Autodesk Fusion 360 part; units mm, degrees
(part 2 of 7)
  line L507 (63.4211, -56.2632) -> (63.3407, -56.2797)
  line L508 (63.3407, -56.2797) -> (63.3132, -56.4089)
  line L509 (63.3132, -56.4089) -> (63.2875, -56.5384)
  line L510 (63.2875, -56.5384) -> (63.2634, -56.6683)
  line L511 (63.2634, -56.6683) -> (63.3314, -56.7143)
  line L512 (63.3314, -56.7143) -> (63.3997, -56.7585)
  line L513 (63.3997, -56.7585) -> (63.4685, -56.801)
  line L514 (63.4685, -56.801) -> (63.5377, -56.8416)
  line L515 (63.5377, -56.8416) -> (63.6073, -56.8801)
  line L516 (63.6073, -56.8801) -> (63.6773, -56.9167)
  line L517 (63.6773, -56.9167) -> (63.7477, -56.951)
  line L518 (63.7477, -56.951) -> (63.8185, -56.9829)
  line L519 (63.8185, -56.9829) -> (63.8898, -57.0123)
  line L520 (63.8898, -57.0123) -> (63.9616, -57.0387)
  line L521 (63.9616, -57.0387) -> (64.0339, -57.0615)
  line L522 (64.0339, -57.0615) -> (64.107, -57.0789)
  line L523 (64.107, -57.0789) -> (64.5136, -57.1395)
  line L524 (64.5136, -57.1395) -> (64.4846, -57.3519)
  line L525 (64.4846, -57.3519) -> (64.461, -57.565)
  line L526 (64.461, -57.565) -> (64.4426, -57.7785)
  line L527 (64.4426, -57.7785) -> (64.4296, -57.9925)
  line L528 (64.4296, -57.9925) -> (64.019, -57.9726)
  line L529 (64.019, -57.9726) -> (63.9439, -57.9754)
  line L530 (63.9439, -57.9754) -> (63.8685, -57.9837)
  line L531 (63.8685, -57.9837) -> (63.793, -57.9956)
  line L532 (63.793, -57.9956) -> (63.7173, -58.0105)
  line L533 (63.7173, -58.0105) -> (63.6416, -58.028)
  line L534 (63.6416, -58.028) -> (63.5659, -58.0479)
  line L535 (63.5659, -58.0479) -> (63.4901, -58.0701)
  line L536 (63.4901, -58.0701) -> (63.4143, -58.0944)
  line L537 (63.4143, -58.0944) -> (63.3385, -58.1207)
  line L538 (63.3385, -58.1207) -> (63.2628, -58.1489)
  line L539 (63.2628, -58.1489) -> (63.1871, -58.1789)
  line L540 (63.1871, -58.1789) -> (63.1115, -58.2108)
  line L541 (63.1115, -58.2108) -> (63.1097, -58.3429)
  line L542 (63.1097, -58.3429) -> (63.1097, -58.4749)
  line L543 (63.1097, -58.4749) -> (63.1115, -58.607)
  line L544 (63.1115, -58.607) -> (63.1871, -58.6389)
  line L545 (63.1871, -58.6389) -> (63.2628, -58.6689)
  line L546 (63.2628, -58.6689) -> (63.3385, -58.6971)
  line L547 (63.3385, -58.6971) -> (63.4143, -58.7234)
  line L548 (63.4143, -58.7234) -> (63.4901, -58.7477)
  line L549 (63.4901, -58.7477) -> (63.5659, -58.7699)
  line L550 (63.5659, -58.7699) -> (63.6416, -58.7898)
  line L551 (63.6416, -58.7898) -> (63.7173, -58.8073)
  line L552 (63.7173, -58.8073) -> (63.793, -58.8222)
  line L553 (63.793, -58.8222) -> (63.8685, -58.8341)
  line L554 (63.8685, -58.8341) -> (63.9439, -58.8424)
  line L555 (63.9439, -58.8424) -> (64.019, -58.8452)
  line L556 (64.019, -58.8452) -> (64.4296, -58.8253)
  line L557 (64.4296, -58.8253) -> (64.4426, -59.0393)
  line L558 (64.4426, -59.0393) -> (64.461, -59.2528)
  line L559 (64.461, -59.2528) -> (64.4846, -59.4659)
  line L560 (64.4846, -59.4659) -> (64.5136, -59.6783)
  line L561 (64.5136, -59.6783) -> (64.107, -59.7389)
  line L562 (64.107, -59.7389) -> (64.0339, -59.7563)
  line L563 (64.0339, -59.7563) -> (63.9616, -59.7791)
  line L564 (63.9616, -59.7791) -> (63.8898, -59.8055)
  line L565 (63.8898, -59.8055) -> (63.8185, -59.8349)
  line L566 (63.8185, -59.8349) -> (63.7477, -59.8668)
  line L567 (63.7477, -59.8668) -> (63.6773, -59.9011)
  line L568 (63.6773, -59.9011) -> (63.6073, -59.9377)
  line L569 (63.6073, -59.9377) -> (63.5377, -59.9762)
  line L570 (63.5377, -59.9762) -> (63.4685, -60.0168)
  line L571 (63.4685, -60.0168) -> (63.3997, -60.0593)
  line L572 (63.3997, -60.0593) -> (63.3314, -60.1035)
  line L573 (63.3314, -60.1035) -> (63.2634, -60.1495)
  line L574 (63.2634, -60.1495) -> (63.2875, -60.2794)
  line L575 (63.2875, -60.2794) -> (63.3132, -60.4089)
  line L576 (63.3132, -60.4089) -> (63.3407, -60.5381)
  line L577 (63.3407, -60.5381) -> (63.4211, -60.5546)
  line L578 (63.4211, -60.5546) -> (63.5012, -60.5693)
  line L579 (63.5012, -60.5693) -> (63.581, -60.5822)
  line L580 (63.581, -60.5822) -> (63.6604, -60.5932)
  line L581 (63.6604, -60.5932) -> (63.7395, -60.6022)
  line L582 (63.7395, -60.6022) -> (63.8181, -60.6092)
  line L583 (63.8181, -60.6092) -> (63.8963, -60.614)
  line L584 (63.8963, -60.614) -> (63.974, -60.6164)
  line L585 (63.974, -60.6164) -> (64.0511, -60.6162)
  line L586 (64.0511, -60.6162) -> (64.1275, -60.6131)
  line L587 (64.1275, -60.6131) -> (64.203, -60.6065)
  line L588 (64.203, -60.6065) -> (64.2773, -60.5947)
  line L589 (64.2773, -60.5947) -> (64.6761, -60.4951)
  line L590 (64.6761, -60.4951) -> (64.7306, -60.7024)
  line L591 (64.7306, -60.7024) -> (64.7903, -60.9083)
  line L592 (64.7903, -60.9083) -> (64.855, -61.1126)
  line L593 (64.855, -61.1126) -> (64.9249, -61.3152)
  line L594 (64.9249, -61.3152) -> (64.538, -61.454)
  line L595 (64.538, -61.454) -> (64.4696, -61.4854)
  line L596 (64.4696, -61.4854) -> (64.4031, -61.5218)
  line L597 (64.4031, -61.5218) -> (64.3379, -61.5617)
  line L598 (64.3379, -61.5617) -> (64.2737, -61.6044)
  line L599 (64.2737, -61.6044) -> (64.2105, -61.6496)
  line L600 (64.2105, -61.6496) -> (64.1481, -61.697)
  line L601 (64.1481, -61.697) -> (64.0866, -61.7465)
  line L602 (64.0866, -61.7465) -> (64.0259, -61.7979)
  line L603 (64.0259, -61.7979) -> (63.9659, -61.8512)
  line L604 (63.9659, -61.8512) -> (63.9067, -61.9062)
  line L605 (63.9067, -61.9062) -> (63.8483, -61.963)
  line L606 (63.8483, -61.963) -> (63.7907, -62.0214)
  line L607 (63.7907, -62.0214) -> (63.8396, -62.144)
  line L608 (63.8396, -62.144) -> (63.8901, -62.266)
  line L609 (63.8901, -62.266) -> (63.9423, -62.3874)
  line L610 (63.9423, -62.3874) -> (64.0243, -62.3879)
  line L611 (64.0243, -62.3879) -> (64.1058, -62.3867)
  line L612 (64.1058, -62.3867) -> (64.1865, -62.3838)
  line L613 (64.1865, -62.3838) -> (64.2666, -62.3791)
  line L614 (64.2666, -62.3791) -> (64.3459, -62.3725)
  line L615 (64.3459, -62.3725) -> (64.4244, -62.364)
  line L616 (64.4244, -62.364) -> (64.502, -62.3534)
  line L617 (64.502, -62.3534) -> (64.5787, -62.3406)
  line L618 (64.5787, -62.3406) -> (64.6542, -62.3254)
  line L619 (64.6542, -62.3254) -> (64.7286, -62.3075)
  line L620 (64.7286, -62.3075) -> (64.8014, -62.2863)
  line L621 (64.8014, -62.2863) -> (64.8719, -62.2601)
  line L622 (64.8719, -62.2601) -> (65.2436, -62.0847)
  line L623 (65.2436, -62.0847) -> (65.3375, -62.2773)
  line L624 (65.3375, -62.2773) -> (65.4362, -62.4676)
  line L625 (65.4362, -62.4676) -> (65.5396, -62.6554)
  line L626 (65.5396, -62.6554) -> (65.6476, -62.8405)
  line L627 (65.6476, -62.8405) -> (65.2952, -63.0521)
  line L628 (65.2952, -63.0521) -> (65.2343, -63.0962)
  line L629 (65.2343, -63.0962) -> (65.1762, -63.145)
  line L630 (65.1762, -63.145) -> (65.12, -63.1968)
  line L631 (65.12, -63.1968) -> (65.0654, -63.2512)
  line L632 (65.0654, -63.2512) -> (65.0122, -63.3078)
  line L633 (65.0122, -63.3078) -> (64.9602, -63.3665)
  line L634 (64.9602, -63.3665) -> (64.9096, -63.427)
  line L635 (64.9096, -63.427) -> (64.86, -63.4893)
  line L636 (64.86, -63.4893) -> (64.8116, -63.5532)
  line L637 (64.8116, -63.5532) -> (64.7643, -63.6188)
  line L638 (64.7643, -63.6188) -> (64.7181, -63.6858)
  line L639 (64.7181, -63.6858) -> (64.6729, -63.7544)
  line L640 (64.6729, -63.7544) -> (64.7448, -63.8651)
  line L641 (64.7448, -63.8651) -> (64.8182, -63.9749)
  line L642 (64.8182, -63.9749) -> (64.893, -64.0838)
  line L643 (64.893, -64.0838) -> (64.9736, -64.0683)
  line L644 (64.9736, -64.0683) -> (65.0533, -64.0512)
  line L645 (65.0533, -64.0512) -> (65.1319, -64.0326)
  line L646 (65.1319, -64.0326) -> (65.2095, -64.0123)
  line L647 (65.2095, -64.0123) -> (65.286, -63.9904)
  line L648 (65.286, -63.9904) -> (65.3613, -63.9667)
  line L649 (65.3613, -63.9667) -> (65.4354, -63.9412)
  line L650 (65.4354, -63.9412) -> (65.5081, -63.9137)
  line L651 (65.5081, -63.9137) -> (65.5792, -63.8841)
  line L652 (65.5792, -63.8841) -> (65.6486, -63.852)
  line L653 (65.6486, -63.852) -> (65.7159, -63.817)
  line L654 (65.7159, -63.817) -> (65.78, -63.7776)
  line L655 (65.78, -63.7776) -> (66.1103, -63.533)
  line L656 (66.1103, -63.533) -> (66.24, -63.7036)
  line L657 (66.24, -63.7036) -> (66.3739, -63.871)
  line L658 (66.3739, -63.871) -> (66.5119, -64.035)
  line L659 (66.5119, -64.035) -> (66.654, -64.1955)
  line L660 (66.654, -64.1955) -> (66.3496, -64.4718)
  line L661 (66.3496, -64.4718) -> (66.2985, -64.5269)
  line L662 (66.2985, -64.5269) -> (66.2511, -64.5861)
  line L663 (66.2511, -64.5861) -> (66.2061, -64.6479)
  line L664 (66.2061, -64.6479) -> (66.1631, -64.7119)
  line L665 (66.1631, -64.7119) -> (66.122, -64.7778)
  line L666 (66.122, -64.7778) -> (66.0825, -64.8455)
  line L667 (66.0825, -64.8455) -> (66.0446, -64.9147)
  line L668 (66.0446, -64.9147) -> (66.0081, -64.9855)
  line L669 (66.0081, -64.9855) -> (65.9731, -65.0576)
  line L670 (65.9731, -65.0576) -> (65.9395, -65.1311)
  line L671 (65.9395, -65.1311) -> (65.9073, -65.2059)
  line L672 (65.9073, -65.2059) -> (65.8764, -65.2819)
  line L673 (65.8764, -65.2819) -> (65.9685, -65.3766)
  line L674 (65.9685, -65.3766) -> (66.0619, -65.4699)
  line L675 (66.0619, -65.4699) -> (66.1565, -65.5621)
  line L676 (66.1565, -65.5621) -> (66.2325, -65.5311)
  line L677 (66.2325, -65.5311) -> (66.3073, -65.4989)
  line L678 (66.3073, -65.4989) -> (66.3808, -65.4653)
  line L679 (66.3808, -65.4653) -> (66.4529, -65.4303)
  line L680 (66.4529, -65.4303) -> (66.5237, -65.3939)
  line L681 (66.5237, -65.3939) -> (66.593, -65.3559)
  line L682 (66.593, -65.3559) -> (66.6606, -65.3165)
  line L683 (66.6606, -65.3165) -> (66.7265, -65.2753)
  line L684 (66.7265, -65.2753) -> (66.7905, -65.2324)
  line L685 (66.7905, -65.2324) -> (66.8524, -65.1874)
  line L686 (66.8524, -65.1874) -> (66.9115, -65.1399)
  line L687 (66.9115, -65.1399) -> (66.9666, -65.0888)
  line L688 (66.9666, -65.0888) -> (67.2429, -64.7844)
  line L689 (67.2429, -64.7844) -> (67.4034, -64.9265)
  line L690 (67.4034, -64.9265) -> (67.5674, -65.0645)
  line L691 (67.5674, -65.0645) -> (67.7348, -65.1984)
  line L692 (67.7348, -65.1984) -> (67.9054, -65.3281)
  line L693 (67.9054, -65.3281) -> (67.6608, -65.6585)
  line L694 (67.6608, -65.6585) -> (67.6214, -65.7225)
  line L695 (67.6214, -65.7225) -> (67.5864, -65.7898)
  line L696 (67.5864, -65.7898) -> (67.5543, -65.8592)
  line L697 (67.5543, -65.8592) -> (67.5247, -65.9303)
  line L698 (67.5247, -65.9303) -> (67.4972, -66.003)
  line L699 (67.4972, -66.003) -> (67.4717, -66.0771)
  line L700 (67.4717, -66.0771) -> (67.448, -66.1524)
  line L701 (67.448, -66.1524) -> (67.4261, -66.2289)
  line L702 (67.4261, -66.2289) -> (67.4058, -66.3065)
  line L703 (67.4058, -66.3065) -> (67.3872, -66.3852)
  line L704 (67.3872, -66.3852) -> (67.3702, -66.4648)
  line L705 (67.3702, -66.4648) -> (67.3547, -66.5454)
  line L706 (67.3547, -66.5454) -> (67.4635, -66.6202)
  line L707 (67.4635, -66.6202) -> (67.5733, -66.6936)
  line L708 (67.5733, -66.6936) -> (67.6841, -66.7655)
  line L709 (67.6841, -66.7655) -> (67.7526, -66.7203)
  line L710 (67.7526, -66.7203) -> (67.8196, -66.6741)
  line L711 (67.8196, -66.6741) -> (67.8852, -66.6268)
  line L712 (67.8852, -66.6268) -> (67.9491, -66.5784)
  line L713 (67.9491, -66.5784) -> (68.0114, -66.5289)
  line L714 (68.0114, -66.5289) -> (68.0719, -66.4782)
  line L715 (68.0719, -66.4782) -> (68.1306, -66.4263)
  line L716 (68.1306, -66.4263) -> (68.1872, -66.373)
  line L717 (68.1872, -66.373) -> (68.2416, -66.3184)
  line L718 (68.2416, -66.3184) -> (68.2935, -66.2622)
  line L719 (68.2935, -66.2622) -> (68.3422, -66.2041)
  line L720 (68.3422, -66.2041) -> (68.3863, -66.1432)
  line L721 (68.3863, -66.1432) -> (68.5979, -65.7908)
  line L722 (68.5979, -65.7908) -> (68.783, -65.8989)
  line L723 (68.783, -65.8989) -> (68.9708, -66.0022)
  line L724 (68.9708, -66.0022) -> (69.1611, -66.1009)
  line L725 (69.1611, -66.1009) -> (69.3538, -66.1948)
  line L726 (69.3538, -66.1948) -> (69.1783, -66.5665)
  line L727 (69.1783, -66.5665) -> (69.1521, -66.6371)
  line L728 (69.1521, -66.6371) -> (69.1309, -66.7099)
  line L729 (69.1309, -66.7099) -> (69.113, -66.7842)
  line L730 (69.113, -66.7842) -> (69.0978, -66.8598)
  line L731 (69.0978, -66.8598) -> (69.085, -66.9364)
  line L732 (69.085, -66.9364) -> (69.0745, -67.014)
  line L733 (69.0745, -67.014) -> (69.0659, -67.0925)
  line L734 (69.0659, -67.0925) -> (69.0594, -67.1718)
  line L735 (69.0594, -67.1718) -> (69.0546, -67.2519)
  line L736 (69.0546, -67.2519) -> (69.0517, -67.3327)
  line L737 (69.0517, -67.3327) -> (69.0505, -67.4141)
  line L738 (69.0505, -67.4141) -> (69.0511, -67.4962)
  line L739 (69.0511, -67.4962) -> (69.1724, -67.5483)
  line L740 (69.1724, -67.5483) -> (69.2944, -67.5989)
  line L741 (69.2944, -67.5989) -> (69.4171, -67.6478)
  line L742 (69.4171, -67.6478) -> (69.4755, -67.5901)
  line L743 (69.4755, -67.5901) -> (69.5322, -67.5317)
  line L744 (69.5322, -67.5317) -> (69.5873, -67.4725)
  line L745 (69.5873, -67.4725) -> (69.6405, -67.4126)
  line L746 (69.6405, -67.4126) -> (69.692, -67.3518)
  line L747 (69.692, -67.3518) -> (69.7414, -67.2903)
  line L748 (69.7414, -67.2903) -> (69.7888, -67.2279)
  line L749 (69.7888, -67.2279) -> (69.834, -67.1647)
  line L750 (69.834, -67.1647) -> (69.8767, -67.1005)
  line L751 (69.8767, -67.1005) -> (69.9166, -67.0353)
  line L752 (69.9166, -67.0353) -> (69.9531, -66.9688)
  line L753 (69.9531, -66.9688) -> (69.9844, -66.9005)
  line L754 (69.9844, -66.9005) -> (70.1232, -66.5135)
  line L755 (70.1232, -66.5135) -> (70.3258, -66.5834)
  line L756 (70.3258, -66.5834) -> (70.5302, -66.6482)
  line L757 (70.5302, -66.6482) -> (70.7361, -66.7078)
  line L758 (70.7361, -66.7078) -> (70.9434, -66.7623)
  line L759 (70.9434, -66.7623) -> (70.8438, -67.1611)
  line L760 (70.8438, -67.1611) -> (70.8319, -67.2354)
  line L761 (70.8319, -67.2354) -> (70.8253, -67.3109)
  line L762 (70.8253, -67.3109) -> (70.8222, -67.3873)
  line L763 (70.8222, -67.3873) -> (70.822, -67.4644)
  line L764 (70.822, -67.4644) -> (70.8245, -67.5421)
  line L765 (70.8245, -67.5421) -> (70.8292, -67.6203)
  line L766 (70.8292, -67.6203) -> (70.8362, -67.6989)
  line L767 (70.8362, -67.6989) -> (70.8452, -67.778)
  line L768 (70.8452, -67.778) -> (70.8562, -67.8574)
  line L769 (70.8562, -67.8574) -> (70.8691, -67.9372)
  line L770 (70.8691, -67.9372) -> (70.8838, -68.0173)
  line L771 (70.8838, -68.0173) -> (70.9003, -68.0977)
  line L772 (70.9003, -68.0977) -> (71.0295, -68.1252)
  line L773 (71.0295, -68.1252) -> (71.159, -68.151)
  line L774 (71.159, -68.151) -> (71.2889, -68.175)
  line L775 (71.2889, -68.175) -> (71.3349, -68.107)
  line L776 (71.3349, -68.107) -> (71.3792, -68.0387)
  line L777 (71.3792, -68.0387) -> (71.4216, -67.9699)
  line L778 (71.4216, -67.9699) -> (71.4622, -67.9007)
  line L779 (71.4622, -67.9007) -> (71.5008, -67.8311)
  line L780 (71.5008, -67.8311) -> (71.5373, -67.7611)
  line L781 (71.5373, -67.7611) -> (71.5716, -67.6907)
  line L782 (71.5716, -67.6907) -> (71.6036, -67.6199)
  line L783 (71.6036, -67.6199) -> (71.6329, -67.5486)
  line L784 (71.6329, -67.5486) -> (71.6593, -67.4768)
  line L785 (71.6593, -67.4768) -> (71.6821, -67.4045)
  line L786 (71.6821, -67.4045) -> (71.6996, -67.3314)
  line L787 (71.6996, -67.3314) -> (71.7602, -66.9248)
  line L788 (71.7602, -66.9248) -> (71.9726, -66.9538)
  line L789 (71.9726, -66.9538) -> (72.1856, -66.9774)
  line L790 (72.1856, -66.9774) -> (72.3992, -66.9958)
  line L791 (72.3992, -66.9958) -> (72.6131, -67.0088)
  line L792 (72.6131, -67.0088) -> (72.5932, -67.4194)
  line L793 (72.5932, -67.4194) -> (72.5961, -67.4945)
  line L794 (72.5961, -67.4945) -> (72.6043, -67.5699)
  line L795 (72.6043, -67.5699) -> (72.6162, -67.6454)
  line L796 (72.6162, -67.6454) -> (72.6311, -67.7211)
  line L797 (72.6311, -67.7211) -> (72.6486, -67.7968)
  line L798 (72.6486, -67.7968) -> (72.6686, -67.8725)
  line L799 (72.6686, -67.8725) -> (72.6907, -67.9483)
  line L800 (72.6907, -67.9483) -> (72.715, -68.0241)
  line L801 (72.715, -68.0241) -> (72.7413, -68.0999)
  line L802 (72.7413, -68.0999) -> (72.7695, -68.1756)
  line L803 (72.7695, -68.1756) -> (72.7996, -68.2513)
  line L804 (72.7996, -68.2513) -> (72.8314, -68.3269)
  line L805 (72.8314, -68.3269) -> (72.9635, -68.3287)
  line L806 (72.9635, -68.3287) -> (73.0956, -68.3287)
  line L807 (73.0956, -68.3287) -> (73.2276, -68.3269)
  line L808 (73.2276, -68.3269) -> (73.2595, -68.2513)
  line L809 (73.2595, -68.2513) -> (73.2896, -68.1756)
  line L810 (73.2896, -68.1756) -> (73.3178, -68.0999)
  line L811 (73.3178, -68.0999) -> (73.3441, -68.0241)
  line L812 (73.3441, -68.0241) -> (73.3683, -67.9483)
  line L813 (73.3683, -67.9483) -> (73.3905, -67.8725)
  line L814 (73.3905, -67.8725) -> (73.4104, -67.7968)
  line L815 (73.4104, -67.7968) -> (73.4279, -67.7211)
  line L816 (73.4279, -67.7211) -> (73.4428, -67.6454)
  line L817 (73.4428, -67.6454) -> (73.4547, -67.5699)
  line L818 (73.4547, -67.5699) -> (73.463, -67.4945)
  line L819 (73.463, -67.4945) -> (73.4658, -67.4194)
  line L820 (73.4658, -67.4194) -> (73.4459, -67.0088)
  line L821 (73.4459, -67.0088) -> (73.6599, -66.9958)
  line L822 (73.6599, -66.9958) -> (73.8734, -66.9774)
  line L823 (73.8734, -66.9774) -> (74.0865, -66.9538)
  line L824 (74.0865, -66.9538) -> (74.2989, -66.9248)
  line L825 (74.2989, -66.9248) -> (74.3595, -67.3314)
  line L826 (74.3595, -67.3314) -> (74.3769, -67.4045)
  line L827 (74.3769, -67.4045) -> (74.3997, -67.4768)
  line L828 (74.3997, -67.4768) -> (74.4261, -67.5486)
  line L829 (74.4261, -67.5486) -> (74.4555, -67.6199)
  line L830 (74.4555, -67.6199) -> (74.4874, -67.6907)
  line L831 (74.4874, -67.6907) -> (74.5218, -67.7611)
  line L832 (74.5218, -67.7611) -> (74.5583, -67.8311)
  line L833 (74.5583, -67.8311) -> (74.5969, -67.9007)
  line L834 (74.5969, -67.9007) -> (74.6374, -67.9699)
  line L835 (74.6374, -67.9699) -> (74.6799, -68.0387)
  line L836 (74.6799, -68.0387) -> (74.7241, -68.107)
  line L837 (74.7241, -68.107) -> (74.7702, -68.175)
  line L838 (74.7702, -68.175) -> (74.9, -68.151)
  line L839 (74.9, -68.151) -> (75.0295, -68.1252)
  line L840 (75.0295, -68.1252) -> (75.1587, -68.0977)
  line L841 (75.1587, -68.0977) -> (75.1752, -68.0173)
  line L842 (75.1752, -68.0173) -> (75.19, -67.9372)
  line L843 (75.19, -67.9372) -> (75.2028, -67.8574)
  line L844 (75.2028, -67.8574) -> (75.2138, -67.778)
  line L845 (75.2138, -67.778) -> (75.2229, -67.6989)
  line L846 (75.2229, -67.6989) -> (75.2298, -67.6203)
  line L847 (75.2298, -67.6203) -> (75.2346, -67.5421)
  line L848 (75.2346, -67.5421) -> (75.237, -67.4644)
  line L849 (75.237, -67.4644) -> (75.2368, -67.3873)
  line L850 (75.2368, -67.3873) -> (75.2338, -67.3109)
  line L851 (75.2338, -67.3109) -> (75.2272, -67.2354)
  line L852 (75.2272, -67.2354) -> (75.2153, -67.1611)
  line L853 (75.2153, -67.1611) -> (75.1157, -66.7623)
  line L854 (75.1157, -66.7623) -> (75.323, -66.7078)
  line L855 (75.323, -66.7078) -> (75.5289, -66.6482)
  line L856 (75.5289, -66.6482) -> (75.7332, -66.5834)
  line L857 (75.7332, -66.5834) -> (75.9359, -66.5135)
  line L858 (75.9359, -66.5135) -> (76.0746, -66.9005)
  line L859 (76.0746, -66.9005) -> (76.106, -66.9688)
  line L860 (76.106, -66.9688) -> (76.1425, -67.0353)
  line L861 (76.1425, -67.0353) -> (76.1824, -67.1005)
  line L862 (76.1824, -67.1005) -> (76.2251, -67.1647)
  line L863 (76.2251, -67.1647) -> (76.2702, -67.2279)
  line L864 (76.2702, -67.2279) -> (76.3176, -67.2903)
  line L865 (76.3176, -67.2903) -> (76.3671, -67.3518)
  line L866 (76.3671, -67.3518) -> (76.4185, -67.4126)
  line L867 (76.4185, -67.4126) -> (76.4718, -67.4725)
  line L868 (76.4718, -67.4725) -> (76.5268, -67.5317)
  line L869 (76.5268, -67.5317) -> (76.5836, -67.5901)
  line L870 (76.5836, -67.5901) -> (76.642, -67.6478)
  line L871 (76.642, -67.6478) -> (76.7647, -67.5989)
  line L872 (76.7647, -67.5989) -> (76.8867, -67.5483)
  line L873 (76.8867, -67.5483) -> (77.008, -67.4962)
  line L874 (77.008, -67.4962) -> (77.0085, -67.4141)
  line L875 (77.0085, -67.4141) -> (77.0073, -67.3327)
  line L876 (77.0073, -67.3327) -> (77.0044, -67.2519)
  line L877 (77.0044, -67.2519) -> (76.9997, -67.1718)
  line L878 (76.9997, -67.1718) -> (76.9931, -67.0925)
  line L879 (76.9931, -67.0925) -> (76.9846, -67.014)
  line L880 (76.9846, -67.014) -> (76.974, -66.9364)
  line L881 (76.974, -66.9364) -> (76.9612, -66.8598)
  line L882 (76.9612, -66.8598) -> (76.946, -66.7842)
  line L883 (76.946, -66.7842) -> (76.9281, -66.7099)
  line L884 (76.9281, -66.7099) -> (76.9069, -66.6371)
  line L885 (76.9069, -66.6371) -> (76.8808, -66.5665)
  line L886 (76.8808, -66.5665) -> (76.7053, -66.1948)
  line L887 (76.7053, -66.1948) -> (76.898, -66.1009)
  line L888 (76.898, -66.1009) -> (77.0882, -66.0022)
  line L889 (77.0882, -66.0022) -> (77.276, -65.8989)
  line L890 (77.276, -65.8989) -> (77.4612, -65.7908)
  line L891 (77.4612, -65.7908) -> (77.6727, -66.1432)
  line L892 (77.6727, -66.1432) -> (77.7168, -66.2041)
  line L893 (77.7168, -66.2041) -> (77.7656, -66.2622)
  line L894 (77.7656, -66.2622) -> (77.8174, -66.3184)
  line L895 (77.8174, -66.3184) -> (77.8718, -66.373)
  line L896 (77.8718, -66.373) -> (77.9285, -66.4263)
  line L897 (77.9285, -66.4263) -> (77.9871, -66.4782)
  line L898 (77.9871, -66.4782) -> (78.0476, -66.5289)
  line L899 (78.0476, -66.5289) -> (78.1099, -66.5784)
  line L900 (78.1099, -66.5784) -> (78.1739, -66.6268)
  line L901 (78.1739, -66.6268) -> (78.2394, -66.6741)
  line L902 (78.2394, -66.6741) -> (78.3065, -66.7203)
  line L903 (78.3065, -66.7203) -> (78.375, -66.7655)
  line L904 (78.375, -66.7655) -> (78.4858, -66.6936)
  line L905 (78.4858, -66.6936) -> (78.5956, -66.6202)
  line L906 (78.5956, -66.6202) -> (78.7044, -66.5454)
  line L907 (78.7044, -66.5454) -> (78.6889, -66.4648)
  line L908 (78.6889, -66.4648) -> (78.6718, -66.3852)
  line L909 (78.6718, -66.3852) -> (78.6532, -66.3065)
  line L910 (78.6532, -66.3065) -> (78.633, -66.2289)
  line L911 (78.633, -66.2289) -> (78.611, -66.1524)
  line L912 (78.611, -66.1524) -> (78.5874, -66.0771)
  line L913 (78.5874, -66.0771) -> (78.5619, -66.003)
  line L914 (78.5619, -66.003) -> (78.5344, -65.9303)
  line L915 (78.5344, -65.9303) -> (78.5047, -65.8592)
  line L916 (78.5047, -65.8592) -> (78.4726, -65.7898)
  line L917 (78.4726, -65.7898) -> (78.4376, -65.7225)
  line L918 (78.4376, -65.7225) -> (78.3982, -65.6585)
  line L919 (78.3982, -65.6585) -> (78.1536, -65.3281)
  line L920 (78.1536, -65.3281) -> (78.3243, -65.1984)
  line L921 (78.3243, -65.1984) -> (78.4916, -65.0645)
  line L922 (78.4916, -65.0645) -> (78.6556, -64.9265)
  line L923 (78.6556, -64.9265) -> (78.8161, -64.7844)
  line L924 (78.8161, -64.7844) -> (79.0924, -65.0888)
  line L925 (79.0924, -65.0888) -> (79.1475, -65.1399)
  line L926 (79.1475, -65.1399) -> (79.2067, -65.1874)
  line L927 (79.2067, -65.1874) -> (79.2685, -65.2324)
  line L928 (79.2685, -65.2324) -> (79.3325, -65.2753)
  line L929 (79.3325, -65.2753) -> (79.3984, -65.3165)
  line L930 (79.3984, -65.3165) -> (79.4661, -65.3559)
  line L931 (79.4661, -65.3559) -> (79.5353, -65.3939)
  line L932 (79.5353, -65.3939) -> (79.6061, -65.4303)
  line L933 (79.6061, -65.4303) -> (79.6783, -65.4653)
  line L934 (79.6783, -65.4653) -> (79.7518, -65.4989)
  line L935 (79.7518, -65.4989) -> (79.8265, -65.5311)
  line L936 (79.8265, -65.5311) -> (79.9026, -65.5621)
  line L937 (79.9026, -65.5621) -> (79.9972, -65.4699)
  line L938 (79.9972, -65.4699) -> (80.0906, -65.3766)
  line L939 (80.0906, -65.3766) -> (80.1827, -65.2819)
  line L940 (80.1827, -65.2819) -> (80.1518, -65.2059)
  line L941 (80.1518, -65.2059) -> (80.1195, -65.1311)
  line L942 (80.1195, -65.1311) -> (80.0859, -65.0576)
  line L943 (80.0859, -65.0576) -> (80.0509, -64.9855)
  line L944 (80.0509, -64.9855) -> (80.0145, -64.9147)
  line L945 (80.0145, -64.9147) -> (79.9766, -64.8455)
  line L946 (79.9766, -64.8455) -> (79.9371, -64.7778)
  line L947 (79.9371, -64.7778) -> (79.8959, -64.7119)
  line L948 (79.8959, -64.7119) -> (79.853, -64.6479)
  line L949 (79.853, -64.6479) -> (79.808, -64.5861)
  line L950 (79.808, -64.5861) -> (79.7605, -64.5269)
  line L951 (79.7605, -64.5269) -> (79.7094, -64.4718)
  line L952 (79.7094, -64.4718) -> (79.405, -64.1955)
  line L953 (79.405, -64.1955) -> (79.5471, -64.035)
  line L954 (79.5471, -64.035) -> (79.6851, -63.871)
  line L955 (79.6851, -63.871) -> (79.8191, -63.7036)
  line L956 (79.8191, -63.7036) -> (79.9488, -63.533)
  line L957 (79.9488, -63.533) -> (80.2791, -63.7776)
  line L958 (80.2791, -63.7776) -> (80.3431, -63.817)
  line L959 (80.3431, -63.817) -> (80.4104, -63.852)
  line L960 (80.4104, -63.852) -> (80.4798, -63.8841)
  line L961 (80.4798, -63.8841) -> (80.551, -63.9137)
  line L962 (80.551, -63.9137) -> (80.6237, -63.9412)
  line L963 (80.6237, -63.9412) -> (80.6977, -63.9667)
  line L964 (80.6977, -63.9667) -> (80.773, -63.9904)
  line L965 (80.773, -63.9904) -> (80.8495, -64.0123)
  line L966 (80.8495, -64.0123) -> (80.9271, -64.0326)
  line L967 (80.9271, -64.0326) -> (81.0058, -64.0512)
  line L968 (81.0058, -64.0512) -> (81.0854, -64.0683)
  line L969 (81.0854, -64.0683) -> (81.166, -64.0838)
  line L970 (81.166, -64.0838) -> (81.2408, -63.9749)
  line L971 (81.2408, -63.9749) -> (81.3142, -63.8651)
  line L972 (81.3142, -63.8651) -> (81.3861, -63.7544)
  line L973 (81.3861, -63.7544) -> (81.3409, -63.6858)
  line L974 (81.3409, -63.6858) -> (81.2947, -63.6188)
  line L975 (81.2947, -63.6188) -> (81.2474, -63.5532)
  line L976 (81.2474, -63.5532) -> (81.199, -63.4893)
  line L977 (81.199, -63.4893) -> (81.1495, -63.427)
  line L978 (81.1495, -63.427) -> (81.0988, -63.3665)
  line L979 (81.0988, -63.3665) -> (81.0469, -63.3078)
  line L980 (81.0469, -63.3078) -> (80.9937, -63.2512)
  line L981 (80.9937, -63.2512) -> (80.939, -63.1968)
  line L982 (80.939, -63.1968) -> (80.8828, -63.145)
  line L983 (80.8828, -63.145) -> (80.8248, -63.0962)
  line L984 (80.8248, -63.0962) -> (80.7639, -63.0521)
  line L985 (80.7639, -63.0521) -> (80.4114, -62.8405)
  line L986 (80.4114, -62.8405) -> (80.5195, -62.6554)
  line L987 (80.5195, -62.6554) -> (80.6229, -62.4676)
  line L988 (80.6229, -62.4676) -> (80.7215, -62.2773)
  line L989 (80.7215, -62.2773) -> (80.8155, -62.0847)
  line L990 (80.8155, -62.0847) -> (81.1872, -62.2601)
  line L991 (81.1872, -62.2601) -> (81.2577, -62.2863)
  line L992 (81.2577, -62.2863) -> (81.3305, -62.3075)
  line L993 (81.3305, -62.3075) -> (81.4048, -62.3254)
  line L994 (81.4048, -62.3254) -> (81.4804, -62.3406)
  line L995 (81.4804, -62.3406) -> (81.557, -62.3534)
  line L996 (81.557, -62.3534) -> (81.6347, -62.364)
  line L997 (81.6347, -62.364) -> (81.7131, -62.3725)
  line L998 (81.7131, -62.3725) -> (81.7924, -62.3791)
  line L999 (81.7924, -62.3791) -> (81.8725, -62.3838)
  line L1000 (81.8725, -62.3838) -> (81.9533, -62.3867)
  line L1001 (81.9533, -62.3867) -> (82.0347, -62.3879)
  line L1002 (82.0347, -62.3879) -> (82.1168, -62.3874)
  line L1003 (82.1168, -62.3874) -> (82.1689, -62.266)
  line L1004 (82.1689, -62.266) -> (82.2195, -62.144)
  line L1005 (82.2195, -62.144) -> (82.2684, -62.0214)
  line L1006 (82.2684, -62.0214) -> (82.2107, -61.963)
  line L1007 (82.2107, -61.963) -> (82.1523, -61.9062)
  line L1008 (82.1523, -61.9062) -> (82.0931, -61.8512)
  line L1009 (82.0931, -61.8512) -> (82.0332, -61.7979)
  line L1010 (82.0332, -61.7979) -> (81.9725, -61.7465)
  line L1011 (81.9725, -61.7465) -> (81.9109, -61.697)
  line L1012 (81.9109, -61.697) -> (81.8486, -61.6496)
  line L1013 (81.8486, -61.6496) -> (81.7853, -61.6044)
  line L1014 (81.7853, -61.6044) -> (81.7211, -61.5617)
  line L1015 (81.7211, -61.5617) -> (81.6559, -61.5218)
  line L1016 (81.6559, -61.5218) -> (81.5894, -61.4854)
  line L1017 (81.5894, -61.4854) -> (81.5211, -61.454)
  line L1018 (81.5211, -61.454) -> (81.1342, -61.3152)
  line L1019 (81.1342, -61.3152) -> (81.204, -61.1126)
  line L1020 (81.204, -61.1126) -> (81.2688, -60.9083)
  line L1021 (81.2688, -60.9083) -> (81.3284, -60.7024)
  line L1022 (81.3284, -60.7024) -> (81.383, -60.4951)
  line L1023 (81.383, -60.4951) -> (81.7818, -60.5947)
  line L1024 (81.7818, -60.5947) -> (81.856, -60.6065)
  line L1025 (81.856, -60.6065) -> (81.9316, -60.6131)
  line L1026 (81.9316, -60.6131) -> (82.008, -60.6162)
  line L1027 (82.008, -60.6162) -> (82.085, -60.6164)
  line L1028 (82.085, -60.6164) -> (82.1627, -60.614)
  line L1029 (82.1627, -60.614) -> (82.2409, -60.6092)
  line L1030 (82.2409, -60.6092) -> (82.3195, -60.6022)
  line L1031 (82.3195, -60.6022) -> (82.3986, -60.5932)
  line L1032 (82.3986, -60.5932) -> (82.4781, -60.5822)
  line L1033 (82.4781, -60.5822) -> (82.5578, -60.5693)
  line L1034 (82.5578, -60.5693) -> (82.6379, -60.5546)
  line L1035 (82.6379, -60.5546) -> (82.7183, -60.5381)
  line L1036 (82.7183, -60.5381) -> (82.7458, -60.4089)
  line L1037 (82.7458, -60.4089) -> (82.7716, -60.2794)
  line L1038 (82.7716, -60.2794) -> (82.7956, -60.1495)
  line L1039 (82.7956, -60.1495) -> (82.7277, -60.1035)
  line L1040 (82.7277, -60.1035) -> (82.6593, -60.0593)
  line L1041 (82.6593, -60.0593) -> (82.5905, -60.0168)
  line L1042 (82.5905, -60.0168) -> (82.5213, -59.9762)
  line L1043 (82.5213, -59.9762) -> (82.4517, -59.9377)
  line L1044 (82.4517, -59.9377) -> (82.3817, -59.9011)
  line L1045 (82.3817, -59.9011) -> (82.3113, -59.8668)
  line L1046 (82.3113, -59.8668) -> (82.2405, -59.8349)
  line L1047 (82.2405, -59.8349) -> (82.1692, -59.8055)
  line L1048 (82.1692, -59.8055) -> (82.0975, -59.7791)
  line L1049 (82.0975, -59.7791) -> (82.0251, -59.7563)
  line L1050 (82.0251, -59.7563) -> (81.952, -59.7389)
  line L1051 (81.952, -59.7389) -> (81.5454, -59.6783)
  line L1052 (81.5454, -59.6783) -> (81.5744, -59.4659)
  line L1053 (81.5744, -59.4659) -> (81.5981, -59.2528)
  line L1054 (81.5981, -59.2528) -> (81.6164, -59.0393)
  line L1055 (81.6164, -59.0393) -> (81.6294, -58.8253)
  circle A0 centre (73.0295, -58.4089) radius 2.2
extrude "Extrude1'" add sketch "Sketch1 (2)" along normal blind 2 separate body makes body 2 in component "CT idler 1"
ref_plane "WorkPlane2" through (0, 0, 39) normal (0, 0, 1) x (1, 0, 0) in component "CT idler 1"
sketch "Sketch2" plane through (0, 0, 39) normal (0, 0, 1) x (1, 0, 0) in component "CT idler 1"
  line L0 (76.0836, -58.8789) -> (76.373, -58.9235)
  line L1 (76.373, -58.9235) -> (76.4443, -58.9246)
  line L2 (76.4443, -58.9246) -> (76.5167, -58.9175)
  line L3 (76.5167, -58.9175) -> (76.5898, -58.9046)
  line L4 (76.5898, -58.9046) -> (76.6635, -58.8869)
  line L5 (76.6635, -58.8869) -> (76.7375, -58.8648)
  line L6 (76.7375, -58.8648) -> (76.8116, -58.8385)
  line L7 (76.8116, -58.8385) -> (76.8859, -58.8084)
  line L8 (76.8859, -58.8084) -> (76.9602, -58.7745)
  line L9 (76.9602, -58.7745) -> (77.0343, -58.7369)
  line L10 (77.0343, -58.7369) -> (77.1083, -58.6958)
  line L11 (77.1083, -58.6958) -> (77.1819, -58.6513)
  line L12 (77.1819, -58.6513) -> (77.2551, -58.6033)
  line L13 (77.2551, -58.6033) -> (77.259, -58.4737)
  line L14 (77.259, -58.4737) -> (77.259, -58.3441)
  line L15 (77.259, -58.3441) -> (77.2551, -58.2145)
  line L16 (77.2551, -58.2145) -> (77.1819, -58.1665)
  line L17 (77.1819, -58.1665) -> (77.1083, -58.122)
  line L18 (77.1083, -58.122) -> (77.0343, -58.0809)
  line L19 (77.0343, -58.0809) -> (76.9602, -58.0433)
  line L20 (76.9602, -58.0433) -> (76.8859, -58.0094)
  line L21 (76.8859, -58.0094) -> (76.8116, -57.9793)
  line L22 (76.8116, -57.9793) -> (76.7375, -57.953)
  line L23 (76.7375, -57.953) -> (76.6635, -57.9309)
  line L24 (76.6635, -57.9309) -> (76.5898, -57.9132)
  line L25 (76.5898, -57.9132) -> (76.5167, -57.9003)
  line L26 (76.5167, -57.9003) -> (76.4443, -57.8932)
  line L27 (76.4443, -57.8932) -> (76.373, -57.8943)
  line L28 (76.373, -57.8943) -> (76.0836, -57.9389)
  line L29 (76.0836, -57.9389) -> (76.0534, -57.7731)
  line L30 (76.0534, -57.7731) -> (76.0142, -57.6091)
  line L31 (76.0142, -57.6091) -> (75.9662, -57.4476)
  line L32 (75.9662, -57.4476) -> (75.9094, -57.2889)
  line L33 (75.9094, -57.2889) -> (76.1824, -57.1828)
  line L34 (76.1824, -57.1828) -> (76.2446, -57.1481)
  line L35 (76.2446, -57.1481) -> (76.3038, -57.1057)
  line L36 (76.3038, -57.1057) -> (76.3607, -57.058)
  line L37 (76.3607, -57.058) -> (76.4156, -57.0059)
  line L38 (76.4156, -57.0059) -> (76.4686, -56.9497)
  line L39 (76.4686, -56.9497) -> (76.5197, -56.8899)
  line L40 (76.5197, -56.8899) -> (76.569, -56.8267)
  line L41 (76.569, -56.8267) -> (76.6164, -56.7602)
  line L42 (76.6164, -56.7602) -> (76.6618, -56.6906)
  line L43 (76.6618, -56.6906) -> (76.7053, -56.618)
  line L44 (76.7053, -56.618) -> (76.7467, -56.5426)
  line L45 (76.7467, -56.5426) -> (76.7861, -56.4645)
  line L46 (76.7861, -56.4645) -> (76.7248, -56.3503)
  line L47 (76.7248, -56.3503) -> (76.66, -56.238)
  line L48 (76.66, -56.238) -> (76.5918, -56.1278)
  line L49 (76.5918, -56.1278) -> (76.5044, -56.1228)
  line L50 (76.5044, -56.1228) -> (76.4183, -56.121)
  line L51 (76.4183, -56.121) -> (76.3338, -56.1224)
  line L52 (76.3338, -56.1224) -> (76.2508, -56.127)
  line L53 (76.2508, -56.127) -> (76.1695, -56.1347)
  line L54 (76.1695, -56.1347) -> (76.0901, -56.1458)
  line L55 (76.0901, -56.1458) -> (76.0128, -56.1601)
  line L56 (76.0128, -56.1601) -> (75.9376, -56.178)
  line L57 (75.9376, -56.178) -> (75.865, -56.1994)
  line L58 (75.865, -56.1994) -> (75.7952, -56.2249)
  line L59 (75.7952, -56.2249) -> (75.7289, -56.2549)
  line L60 (75.7289, -56.2549) -> (75.6678, -56.2915)
  line L61 (75.6678, -56.2915) -> (75.4394, -56.4748)
  line L62 (75.4394, -56.4748) -> (75.3304, -56.3463)
  line L63 (75.3304, -56.3463) -> (75.2145, -56.2239)
  line L64 (75.2145, -56.2239) -> (75.0921, -56.1081)
  line L65 (75.0921, -56.1081) -> (74.9636, -55.999)
  line L66 (74.9636, -55.999) -> (75.1469, -55.7706)
  line L67 (75.1469, -55.7706) -> (75.1835, -55.7095)
  line L68 (75.1835, -55.7095) -> (75.2135, -55.6432)
  line L69 (75.2135, -55.6432) -> (75.239, -55.5734)
  line L70 (75.239, -55.5734) -> (75.2604, -55.5008)
  line L71 (75.2604, -55.5008) -> (75.2783, -55.4257)
  line L72 (75.2783, -55.4257) -> (75.2926, -55.3483)
  line L73 (75.2926, -55.3483) -> (75.3037, -55.2689)
  line L74 (75.3037, -55.2689) -> (75.3115, -55.1876)
  line L75 (75.3115, -55.1876) -> (75.316, -55.1047)
  line L76 (75.316, -55.1047) -> (75.3174, -55.0201)
  line L77 (75.3174, -55.0201) -> (75.3156, -54.934)
  line L78 (75.3156, -54.934) -> (75.3106, -54.8467)
  line L79 (75.3106, -54.8467) -> (75.2004, -54.7784)
  line L80 (75.2004, -54.7784) -> (75.0881, -54.7136)
  line L81 (75.0881, -54.7136) -> (74.974, -54.6523)
  line L82 (74.974, -54.6523) -> (74.8958, -54.6917)
  line L83 (74.8958, -54.6917) -> (74.8204, -54.7331)
  line L84 (74.8204, -54.7331) -> (74.7478, -54.7766)
  line L85 (74.7478, -54.7766) -> (74.6782, -54.822)
  line L86 (74.6782, -54.822) -> (74.6118, -54.8694)
  line L87 (74.6118, -54.8694) -> (74.5485, -54.9187)
  line L88 (74.5485, -54.9187) -> (74.4887, -54.9698)
  line L89 (74.4887, -54.9698) -> (74.4326, -55.0228)
  line L90 (74.4326, -55.0228) -> (74.3804, -55.0777)
  line L91 (74.3804, -55.0777) -> (74.3327, -55.1346)
  line L92 (74.3327, -55.1346) -> (74.2903, -55.1938)
  line L93 (74.2903, -55.1938) -> (74.2556, -55.256)
  line L94 (74.2556, -55.256) -> (74.1495, -55.529)
  line L95 (74.1495, -55.529) -> (73.9908, -55.4722)
  line L96 (73.9908, -55.4722) -> (73.8293, -55.4242)
  line L97 (73.8293, -55.4242) -> (73.6654, -55.385)
  line L98 (73.6654, -55.385) -> (73.4996, -55.3549)
  line L99 (73.4996, -55.3549) -> (73.5441, -55.0654)
  line L100 (73.5441, -55.0654) -> (73.5452, -54.9941)
  line L101 (73.5452, -54.9941) -> (73.5381, -54.9217)
  line L102 (73.5381, -54.9217) -> (73.5252, -54.8486)
  line L103 (73.5252, -54.8486) -> (73.5075, -54.7749)
  line L104 (73.5075, -54.7749) -> (73.4854, -54.701)
  line L105 (73.4854, -54.701) -> (73.4591, -54.6268)
  line L106 (73.4591, -54.6268) -> (73.429, -54.5525)
  line L107 (73.429, -54.5525) -> (73.3951, -54.4782)
  line L108 (73.3951, -54.4782) -> (73.3576, -54.4041)
  line L109 (73.3576, -54.4041) -> (73.3165, -54.3302)
  line L110 (73.3165, -54.3302) -> (73.2719, -54.2566)
  line L111 (73.2719, -54.2566) -> (73.2239, -54.1834)
  line L112 (73.2239, -54.1834) -> (73.0943, -54.1794)
  line L113 (73.0943, -54.1794) -> (72.9647, -54.1794)
  line L114 (72.9647, -54.1794) -> (72.8352, -54.1834)
  line L115 (72.8352, -54.1834) -> (72.7872, -54.2566)
  line L116 (72.7872, -54.2566) -> (72.7426, -54.3302)
  line L117 (72.7426, -54.3302) -> (72.7015, -54.4041)
  line L118 (72.7015, -54.4041) -> (72.6639, -54.4782)
  line L119 (72.6639, -54.4782) -> (72.63, -54.5525)
  line L120 (72.63, -54.5525) -> (72.5999, -54.6268)
  line L121 (72.5999, -54.6268) -> (72.5737, -54.701)
  line L122 (72.5737, -54.701) -> (72.5515, -54.7749)
  line L123 (72.5515, -54.7749) -> (72.5338, -54.8486)
  line L124 (72.5338, -54.8486) -> (72.521, -54.9217)
  line L125 (72.521, -54.9217) -> (72.5138, -54.9941)
  line L126 (72.5138, -54.9941) -> (72.5149, -55.0654)
  line L127 (72.5149, -55.0654) -> (72.5595, -55.3549)
  line L128 (72.5595, -55.3549) -> (72.3937, -55.385)
  line L129 (72.3937, -55.385) -> (72.2298, -55.4242)
  line L130 (72.2298, -55.4242) -> (72.0682, -55.4722)
  line L131 (72.0682, -55.4722) -> (71.9096, -55.529)
  line L132 (71.9096, -55.529) -> (71.8034, -55.256)
  line L133 (71.8034, -55.256) -> (71.7688, -55.1938)
  line L134 (71.7688, -55.1938) -> (71.7264, -55.1346)
  line L135 (71.7264, -55.1346) -> (71.6786, -55.0777)
  line L136 (71.6786, -55.0777) -> (71.6265, -55.0228)
  line L137 (71.6265, -55.0228) -> (71.5703, -54.9698)
  line L138 (71.5703, -54.9698) -> (71.5105, -54.9187)
  line L139 (71.5105, -54.9187) -> (71.4473, -54.8694)
  line L140 (71.4473, -54.8694) -> (71.3808, -54.822)
  line L141 (71.3808, -54.822) -> (71.3112, -54.7766)
  line L142 (71.3112, -54.7766) -> (71.2387, -54.7331)
  line L143 (71.2387, -54.7331) -> (71.1632, -54.6917)
  line L144 (71.1632, -54.6917) -> (71.0851, -54.6523)
  line L145 (71.0851, -54.6523) -> (70.9709, -54.7136)
  line L146 (70.9709, -54.7136) -> (70.8586, -54.7784)
  line L147 (70.8586, -54.7784) -> (70.7484, -54.8467)
  line L148 (70.7484, -54.8467) -> (70.7435, -54.934)
  line L149 (70.7435, -54.934) -> (70.7417, -55.0201)
  line L150 (70.7417, -55.0201) -> (70.743, -55.1047)
  line L151 (70.743, -55.1047) -> (70.7476, -55.1876)
  line L152 (70.7476, -55.1876) -> (70.7554, -55.2689)
  line L153 (70.7554, -55.2689) -> (70.7664, -55.3483)
  line L154 (70.7664, -55.3483) -> (70.7808, -55.4257)
  line L155 (70.7808, -55.4257) -> (70.7986, -55.5008)
  line L156 (70.7986, -55.5008) -> (70.8201, -55.5734)
  line L157 (70.8201, -55.5734) -> (70.8455, -55.6432)
  line L158 (70.8455, -55.6432) -> (70.8755, -55.7095)
  line L159 (70.8755, -55.7095) -> (70.9121, -55.7706)
  line L160 (70.9121, -55.7706) -> (71.0954, -55.999)
  line L161 (71.0954, -55.999) -> (70.9669, -56.1081)
  line L162 (70.9669, -56.1081) -> (70.8446, -56.2239)
  line L163 (70.8446, -56.2239) -> (70.7287, -56.3463)
  line L164 (70.7287, -56.3463) -> (70.6197, -56.4748)
  line L165 (70.6197, -56.4748) -> (70.3912, -56.2915)
  line L166 (70.3912, -56.2915) -> (70.3301, -56.2549)
  line L167 (70.3301, -56.2549) -> (70.2638, -56.2249)
  line L168 (70.2638, -56.2249) -> (70.194, -56.1994)
  line L169 (70.194, -56.1994) -> (70.1214, -56.178)
  line L170 (70.1214, -56.178) -> (70.0463, -56.1601)
  line L171 (70.0463, -56.1601) -> (69.9689, -56.1458)
  line L172 (69.9689, -56.1458) -> (69.8895, -56.1347)
  line L173 (69.8895, -56.1347) -> (69.8083, -56.127)
  line L174 (69.8083, -56.127) -> (69.7253, -56.1224)
  line L175 (69.7253, -56.1224) -> (69.6407, -56.121)
  line L176 (69.6407, -56.121) -> (69.5547, -56.1228)
  line L177 (69.5547, -56.1228) -> (69.4673, -56.1278)
  line L178 (69.4673, -56.1278) -> (69.3991, -56.238)
  line L179 (69.3991, -56.238) -> (69.3343, -56.3503)
  line L180 (69.3343, -56.3503) -> (69.2729, -56.4645)
  line L181 (69.2729, -56.4645) -> (69.3123, -56.5426)
  line L182 (69.3123, -56.5426) -> (69.3538, -56.618)
  line L183 (69.3538, -56.618) -> (69.3972, -56.6906)
  line L184 (69.3972, -56.6906) -> (69.4427, -56.7602)
  line L185 (69.4427, -56.7602) -> (69.49, -56.8267)
  line L186 (69.49, -56.8267) -> (69.5393, -56.8899)
  line L187 (69.5393, -56.8899) -> (69.5904, -56.9497)
  line L188 (69.5904, -56.9497) -> (69.6434, -57.0059)
  line L189 (69.6434, -57.0059) -> (69.6983, -57.058)
  line L190 (69.6983, -57.058) -> (69.7552, -57.1057)
  line L191 (69.7552, -57.1057) -> (69.8144, -57.1481)
  line L192 (69.8144, -57.1481) -> (69.8766, -57.1828)
  line L193 (69.8766, -57.1828) -> (70.1496, -57.2889)
  line L194 (70.1496, -57.2889) -> (70.0929, -57.4476)
  line L195 (70.0929, -57.4476) -> (70.0448, -57.6091)
  line L196 (70.0448, -57.6091) -> (70.0056, -57.7731)
  line L197 (70.0056, -57.7731) -> (69.9755, -57.9389)
  line L198 (69.9755, -57.9389) -> (69.686, -57.8943)
  line L199 (69.686, -57.8943) -> (69.6148, -57.8932)
  line L200 (69.6148, -57.8932) -> (69.5423, -57.9003)
  line L201 (69.5423, -57.9003) -> (69.4692, -57.9132)
  line L202 (69.4692, -57.9132) -> (69.3956, -57.9309)
  line L203 (69.3956, -57.9309) -> (69.3216, -57.953)
  line L204 (69.3216, -57.953) -> (69.2474, -57.9793)
  line L205 (69.2474, -57.9793) -> (69.1731, -58.0094)
  line L206 (69.1731, -58.0094) -> (69.0989, -58.0433)
  line L207 (69.0989, -58.0433) -> (69.0247, -58.0809)
  line L208 (69.0247, -58.0809) -> (68.9508, -58.122)
  line L209 (68.9508, -58.122) -> (68.8772, -58.1665)
  line L210 (68.8772, -58.1665) -> (68.804, -58.2145)
  line L211 (68.804, -58.2145) -> (68.8, -58.3441)
  line L212 (68.8, -58.3441) -> (68.8, -58.4737)
  line L213 (68.8, -58.4737) -> (68.804, -58.6033)
  line L214 (68.804, -58.6033) -> (68.8772, -58.6513)
  line L215 (68.8772, -58.6513) -> (68.9508, -58.6958)
  line L216 (68.9508, -58.6958) -> (69.0247, -58.7369)
  line L217 (69.0247, -58.7369) -> (69.0989, -58.7745)
  line L218 (69.0989, -58.7745) -> (69.1731, -58.8084)
  line L219 (69.1731, -58.8084) -> (69.2474, -58.8385)
  line L220 (69.2474, -58.8385) -> (69.3216, -58.8648)
  line L221 (69.3216, -58.8648) -> (69.3956, -58.8869)
  line L222 (69.3956, -58.8869) -> (69.4692, -58.9046)
  line L223 (69.4692, -58.9046) -> (69.5423, -58.9175)
  line L224 (69.5423, -58.9175) -> (69.6148, -58.9246)
  line L225 (69.6148, -58.9246) -> (69.686, -58.9235)
  line L226 (69.686, -58.9235) -> (69.9755, -58.8789)
  line L227 (69.9755, -58.8789) -> (70.0056, -59.0447)
  line L228 (70.0056, -59.0447) -> (70.0448, -59.2086)
  line L229 (70.0448, -59.2086) -> (70.0929, -59.3702)
  line L230 (70.0929, -59.3702) -> (70.1496, -59.5289)
  line L231 (70.1496, -59.5289) -> (69.8766, -59.635)
  line L232 (69.8766, -59.635) -> (69.8144, -59.6697)
  line L233 (69.8144, -59.6697) -> (69.7552, -59.7121)
  line L234 (69.7552, -59.7121) -> (69.6983, -59.7598)
  line L235 (69.6983, -59.7598) -> (69.6434, -59.8119)
  line L236 (69.6434, -59.8119) -> (69.5904, -59.8681)
  line L237 (69.5904, -59.8681) -> (69.5393, -59.9279)
  line L238 (69.5393, -59.9279) -> (69.49, -59.9911)
  line L239 (69.49, -59.9911) -> (69.4427, -60.0576)
  line L240 (69.4427, -60.0576) -> (69.3972, -60.1272)
  line L241 (69.3972, -60.1272) -> (69.3538, -60.1998)
  line L242 (69.3538, -60.1998) -> (69.3123, -60.2752)
  line L243 (69.3123, -60.2752) -> (69.2729, -60.3533)
  line L244 (69.2729, -60.3533) -> (69.3343, -60.4675)
  line L245 (69.3343, -60.4675) -> (69.3991, -60.5798)
  line L246 (69.3991, -60.5798) -> (69.4673, -60.69)
  line L247 (69.4673, -60.69) -> (69.5547, -60.695)
  line L248 (69.5547, -60.695) -> (69.6407, -60.6968)
  line L249 (69.6407, -60.6968) -> (69.7253, -60.6954)
  line L250 (69.7253, -60.6954) -> (69.8083, -60.6908)
  line L251 (69.8083, -60.6908) -> (69.8895, -60.6831)
  line L252 (69.8895, -60.6831) -> (69.9689, -60.672)
  line L253 (69.9689, -60.672) -> (70.0463, -60.6576)
  line L254 (70.0463, -60.6576) -> (70.1214, -60.6398)
  line L255 (70.1214, -60.6398) -> (70.194, -60.6184)
  line L256 (70.194, -60.6184) -> (70.2638, -60.5929)
  line L257 (70.2638, -60.5929) -> (70.3301, -60.5629)
  line L258 (70.3301, -60.5629) -> (70.3912, -60.5263)
  line L259 (70.3912, -60.5263) -> (70.6197, -60.343)
  line L260 (70.6197, -60.343) -> (70.7287, -60.4715)
  line L261 (70.7287, -60.4715) -> (70.8446, -60.5939)
  line L262 (70.8446, -60.5939) -> (70.9669, -60.7097)
  line L263 (70.9669, -60.7097) -> (71.0954, -60.8188)
  line L264 (71.0954, -60.8188) -> (70.9121, -61.0472)
  line L265 (70.9121, -61.0472) -> (70.8755, -61.1083)
  line L266 (70.8755, -61.1083) -> (70.8455, -61.1746)
  line L267 (70.8455, -61.1746) -> (70.8201, -61.2444)
  line L268 (70.8201, -61.2444) -> (70.7986, -61.317)
  line L269 (70.7986, -61.317) -> (70.7808, -61.3921)
  line L270 (70.7808, -61.3921) -> (70.7664, -61.4695)
  line L271 (70.7664, -61.4695) -> (70.7554, -61.5489)
  line L272 (70.7554, -61.5489) -> (70.7476, -61.6302)
  line L273 (70.7476, -61.6302) -> (70.743, -61.7131)
  line L274 (70.743, -61.7131) -> (70.7417, -61.7977)
  line L275 (70.7417, -61.7977) -> (70.7435, -61.8838)
  line L276 (70.7435, -61.8838) -> (70.7484, -61.9711)
  line L277 (70.7484, -61.9711) -> (70.8586, -62.0394)
  line L278 (70.8586, -62.0394) -> (70.9709, -62.1042)
  line L279 (70.9709, -62.1042) -> (71.0851, -62.1655)
  line L280 (71.0851, -62.1655) -> (71.1632, -62.1261)
  line L281 (71.1632, -62.1261) -> (71.2387, -62.0847)
  line L282 (71.2387, -62.0847) -> (71.3112, -62.0412)
  line L283 (71.3112, -62.0412) -> (71.3808, -61.9957)
  line L284 (71.3808, -61.9957) -> (71.4473, -61.9484)
  line L285 (71.4473, -61.9484) -> (71.5105, -61.8991)
  line L286 (71.5105, -61.8991) -> (71.5703, -61.848)
  line L287 (71.5703, -61.848) -> (71.6265, -61.795)
  line L288 (71.6265, -61.795) -> (71.6786, -61.7401)
  line L289 (71.6786, -61.7401) -> (71.7264, -61.6832)
  line L290 (71.7264, -61.6832) -> (71.7688, -61.624)
  line L291 (71.7688, -61.624) -> (71.8034, -61.5618)
  line L292 (71.8034, -61.5618) -> (71.9096, -61.2888)
  line L293 (71.9096, -61.2888) -> (72.0682, -61.3456)
  line L294 (72.0682, -61.3456) -> (72.2298, -61.3936)
  line L295 (72.2298, -61.3936) -> (72.3937, -61.4328)
  line L296 (72.3937, -61.4328) -> (72.5595, -61.4629)
  line L297 (72.5595, -61.4629) -> (72.5149, -61.7524)
  line L298 (72.5149, -61.7524) -> (72.5138, -61.8237)
  line L299 (72.5138, -61.8237) -> (72.521, -61.8961)
  line L300 (72.521, -61.8961) -> (72.5338, -61.9692)
  line L301 (72.5338, -61.9692) -> (72.5515, -62.0429)
  line L302 (72.5515, -62.0429) -> (72.5737, -62.1168)
  line L303 (72.5737, -62.1168) -> (72.5999, -62.191)
  line L304 (72.5999, -62.191) -> (72.63, -62.2653)
  line L305 (72.63, -62.2653) -> (72.6639, -62.3396)
  line L306 (72.6639, -62.3396) -> (72.7015, -62.4137)
  line L307 (72.7015, -62.4137) -> (72.7426, -62.4876)
  line L308 (72.7426, -62.4876) -> (72.7872, -62.5612)
  line L309 (72.7872, -62.5612) -> (72.8352, -62.6344)
  line L310 (72.8352, -62.6344) -> (72.9647, -62.6384)
  line L311 (72.9647, -62.6384) -> (73.0943, -62.6384)
  line L312 (73.0943, -62.6384) -> (73.2239, -62.6344)
  line L313 (73.2239, -62.6344) -> (73.2719, -62.5612)
  line L314 (73.2719, -62.5612) -> (73.3165, -62.4876)
  line L315 (73.3165, -62.4876) -> (73.3576, -62.4137)
  line L316 (73.3576, -62.4137) -> (73.3951, -62.3396)
  line L317 (73.3951, -62.3396) -> (73.429, -62.2653)
  line L318 (73.429, -62.2653) -> (73.4591, -62.191)
  line L319 (73.4591, -62.191) -> (73.4854, -62.1168)
  line L320 (73.4854, -62.1168) -> (73.5075, -62.0429)
  line L321 (73.5075, -62.0429) -> (73.5252, -61.9692)
  line L322 (73.5252, -61.9692) -> (73.5381, -61.8961)
  line L323 (73.5381, -61.8961) -> (73.5452, -61.8237)
  line L324 (73.5452, -61.8237) -> (73.5441, -61.7524)
  line L325 (73.5441, -61.7524) -> (73.4996, -61.4629)
  line L326 (73.4996, -61.4629) -> (73.6654, -61.4328)
  line L327 (73.6654, -61.4328) -> (73.8293, -61.3936)
  line L328 (73.8293, -61.3936) -> (73.9908, -61.3456)
  line L329 (73.9908, -61.3456) -> (74.1495, -61.2888)
  line L330 (74.1495, -61.2888) -> (74.2556, -61.5618)
  line L331 (74.2556, -61.5618) -> (74.2903, -61.624)
  line L332 (74.2903, -61.624) -> (74.3327, -61.6832)
  line L333 (74.3327, -61.6832) -> (74.3804, -61.7401)
  line L334 (74.3804, -61.7401) -> (74.4326, -61.795)
  line L335 (74.4326, -61.795) -> (74.4887, -61.848)
  line L336 (74.4887, -61.848) -> (74.5485, -61.8991)
  line L337 (74.5485, -61.8991) -> (74.6118, -61.9484)
  line L338 (74.6118, -61.9484) -> (74.6782, -61.9957)
  line L339 (74.6782, -61.9957) -> (74.7478, -62.0412)
  line L340 (74.7478, -62.0412) -> (74.8204, -62.0847)
  line L341 (74.8204, -62.0847) -> (74.8958, -62.1261)
  line L342 (74.8958, -62.1261) -> (74.974, -62.1655)
  line L343 (74.974, -62.1655) -> (75.0881, -62.1042)
  line L344 (75.0881, -62.1042) -> (75.2004, -62.0394)
  line L345 (75.2004, -62.0394) -> (75.3106, -61.9711)
  line L346 (75.3106, -61.9711) -> (75.3156, -61.8838)
  line L347 (75.3156, -61.8838) -> (75.3174, -61.7977)
  line L348 (75.3174, -61.7977) -> (75.316, -61.7131)
  line L349 (75.316, -61.7131) -> (75.3115, -61.6302)
  line L350 (75.3115, -61.6302) -> (75.3037, -61.5489)
  line L351 (75.3037, -61.5489) -> (75.2926, -61.4695)
  line L352 (75.2926, -61.4695) -> (75.2783, -61.3921)
  line L353 (75.2783, -61.3921) -> (75.2604, -61.317)
  line L354 (75.2604, -61.317) -> (75.239, -61.2444)
  line L355 (75.239, -61.2444) -> (75.2135, -61.1746)
  line L356 (75.2135, -61.1746) -> (75.1835, -61.1083)
  line L357 (75.1835, -61.1083) -> (75.1469, -61.0472)
  line L358 (75.1469, -61.0472) -> (74.9636, -60.8188)
  line L359 (74.9636, -60.8188) -> (75.0921, -60.7097)